Back Cover (Autodesk Fusion 360 design; units mm, degrees)
Autodesk Fusion 360 part; units mm, degrees
sketch "Sketch1" plane through (0, 0, 0) normal (0, 0, 1) x (1, 0, 0)
  line L0 (-79.25, 60.9) -> (79.25, 60.9)
  line L1 (79.25, 60.9) -> (79.25, -60.9)
  line L2 (79.25, -60.9) -> (-79.25, -60.9)
  line L3 (-79.25, -60.9) -> (-79.25, 60.9)
  line L4 (-79.25, 60.9) -> (79.25, -60.9) construction
  line L5 (79.25, 60.9) -> (-79.25, -60.9) construction
  line L6 (79.25, -40.9) -> (-79.25, -40.9)
  line L7 (-79.25, -40.9) -> (-79.25, 40.9)
  line L8 (-79.25, 40.9) -> (79.25, 40.9)
  line L9 (79.25, 40.9) -> (79.25, -40.9)
  line L10 (79.25, -40.9) -> (-79.25, 40.9) construction
  line L11 (-79.25, -40.9) -> (79.25, 40.9) construction
  line L12 (0, 0) -> (0, 60.9) construction
  line L13 (-79.25, 60.9) -> (79.25, 40.9) construction
  line L14 (0, 50.9) -> (-79.25, 50.9) construction
  line L15 (0, 50.9) -> (79.25, 50.9) construction
  line L16 (-2.1, 52.15) -> (-2.1, 49.65)
  arc A0 (-2.1, 49.65) -> (2.1, 49.65) centre (0, 49.65) ccw
  line L17 (2.1, 49.65) -> (2.1, 52.15)
  arc A1 (2.1, 52.15) -> (-2.1, 52.15) centre (0, 52.15) ccw
  line L18 (0, 52.15) -> (0, 49.65) construction
  arc A2 (-50.7333, 52.15) -> (-54.9333, 52.15) centre (-52.8333, 52.15) ccw
  line L19 (-54.9333, 52.15) -> (-54.9333, 49.65)
  arc A3 (-54.9333, 49.65) -> (-50.7333, 49.65) centre (-52.8333, 49.65) ccw
  line L20 (-50.7333, 49.65) -> (-50.7333, 52.15)
  arc A4 (54.9333, 52.15) -> (50.7333, 52.15) centre (52.8333, 52.15) ccw
  line L21 (50.7333, 52.15) -> (50.7333, 49.65)
  arc A5 (50.7333, 49.65) -> (54.9333, 49.65) centre (52.8333, 49.65) ccw
  line L22 (54.9333, 49.65) -> (54.9333, 52.15)
  line L23 (-79.25, 0) -> (79.25, 0) construction
  arc A6 (-54.9333, -52.15) -> (-50.7333, -52.15) centre (-52.8333, -52.15) ccw
  line L24 (-54.9333, -52.15) -> (-54.9333, -49.65)
  arc A7 (-50.7333, -49.65) -> (-54.9333, -49.65) centre (-52.8333, -49.65) ccw
  line L25 (-50.7333, -49.65) -> (-50.7333, -52.15)
  arc A8 (-2.1, -52.15) -> (2.1, -52.15) centre (0, -52.15) ccw
  line L26 (-2.1, -52.15) -> (-2.1, -49.65)
  line L27 (2.1, -49.65) -> (2.1, -52.15)
  arc A9 (2.1, -49.65) -> (-2.1, -49.65) centre (0, -49.65) ccw
  arc A10 (50.7333, -52.15) -> (54.9333, -52.15) centre (52.8333, -52.15) ccw
  line L28 (50.7333, -52.15) -> (50.7333, -49.65)
  line L29 (54.9333, -49.65) -> (54.9333, -52.15)
  arc A11 (54.9333, -49.65) -> (50.7333, -49.65) centre (52.8333, -49.65) ccw
  line L30 (-2.1, 50.9) -> (2.1, 50.9) construction
  line L31 (-37.25, 40.9) -> (-37.25, -40.9) construction
  line L32 (-40.25, 15) -> (-76.25, 15)
  line L33 (-76.25, 15) -> (-76.25, -15)
  line L34 (-76.25, -15) -> (-40.25, -15)
  line L35 (-40.25, -15) -> (-40.25, 15)
  line L36 (-40.25, 15) -> (-76.25, -15) construction
  line L37 (-76.25, 15) -> (-40.25, -15) construction
  line L38 (-43.25, -30) -> (-73.25, -30) construction
  line L39 (-73.25, -30) -> (-73.25, 30) construction
  line L40 (-73.25, 30) -> (-43.25, 30) construction
  line L41 (-43.25, 30) -> (-43.25, -30) construction
  line L42 (-43.25, -30) -> (-73.25, 30) construction
  line L43 (-73.25, -30) -> (-43.25, 30) construction
  circle A12 centre (-73.25, -30) radius 2.1
  circle A13 centre (-43.25, -30) radius 2.1
  circle A14 centre (-73.25, 30) radius 2.1
  circle A15 centre (-43.25, 30) radius 2.1
  line L44 (-79.25, 60.9) -> (-82.25, 60.9)
  line L45 (-82.25, 60.9) -> (-82.25, -60.9)
  line L46 (-82.25, -60.9) -> (-79.25, -60.9)
  line L47 (-79.25, -60.9) -> (-79.25, 60.9)
  point P0 (-58.25, 0)
  point P1 (-58.25, 0)
  dimension "d1" = 121.8
  dimension "d2" = 158.5
  dimension "d3" = 81.8
  dimension "d13" = 4.2
  dimension "d14" = 2.5
  dimension "d22" = 52.8333
  dimension "d23" = 0
  dimension "d26" = 42
  dimension "d27" = 36
  dimension "d28" = 30
  dimension "d29" = 3
  dimension "d30" = 30
  dimension "d31" = 60
  dimension "d32" = 4.2
  dimension "d33" = 4.2
  dimension "d34" = 4.2
  dimension "d35" = 4.2
  dimension "d40" = 3
  constraint perpendicular L0 L1
  constraint parallel L0 L2
  constraint perpendicular L6 L7
  constraint parallel L6 L8
  constraint horizontal L6
  constraint coincident L1 L6.start
  constraint midpoint L0 L12.end
  constraint midpoint L13 L14.start
  constraint coincident L3 L14.end
  constraint perpendicular L3 L14
  constraint coincident L1 L15.end
  constraint perpendicular L1 L15
  constraint tangent L16 A0
  constraint tangent A0 L17
  constraint parallel L16 L17
  constraint tangent L17 A1
  constraint tangent L16 A1
  constraint perpendicular L14 L18
  constraint coincident L12.start L4
  constraint midpoint L12.start L4
  constraint midpoint L12.start L5
  constraint midpoint L12.start L10
  constraint midpoint L12.start L11
  constraint coincident L12.start origin
  constraint coincident L12 A1.centre
  constraint midpoint L3 L23.start
  constraint midpoint L1 L23.end
  constraint symmetric L16.start L23 A8.start
  constraint symmetric L16.end L23 L26.end
  constraint symmetric A0.end L23 L27.start
  constraint symmetric L17.end L23 A8.end
  constraint symmetric A0 L23 A9
  constraint symmetric A1 L23 A8
  constraint symmetric A2.start L23 A6.end
  constraint symmetric A2.end L23 A6.start
  constraint symmetric A2 L23 A6
  constraint symmetric L19.end L23 L24.end
  constraint symmetric A3.end L23 A7.start
  constraint symmetric A3 L23 A7
  constraint symmetric A4.start L23 A10.end
  constraint symmetric A4.end L23 A10.start
  constraint symmetric A4 L23 A10
  constraint symmetric L21.end L23 L28.end
  constraint symmetric A5.end L23 L29.start
  constraint symmetric A5 L23 A11
  constraint midpoint L16 L30.start
  constraint midpoint L17 L30.end
  constraint coincident L14.start L30
  constraint coincident L8 L31.start
  constraint coincident L6 L31.end
  constraint perpendicular L6 L31
  constraint horizontal L32
  constraint perpendicular L32 L33
  constraint parallel L32 L34
  constraint parallel L33 L35
  constraint coincident L36 P1
  constraint coincident L37 P1
  constraint coincident L23 P1
  constraint horizontal L38
  constraint perpendicular L38 L39
  constraint parallel L38 L40
  constraint parallel L39 L41
  constraint coincident L42 P1
  constraint coincident L43 P1
  constraint coincident P1 P0
  constraint coincident L38.end L39.start
  constraint coincident L38.start L41.end
  constraint coincident L39.end L40.start
  constraint coincident L40.end L41.start
  constraint horizontal L44
  constraint vertical L45
  constraint horizontal L46
  constraint vertical L47
  constraint coincident L2.end L3.start
  measures "d1" distance of L0.start L2.end
  measures "d2" distance of L0.start L0.end
  measures "d3" distance of L6.end L7.end
  measures "d13" diameter of A0
  measures "d14" distance of A1.centre A0.centre
  measures "d26" distance of L3 L31
  measures "d27" distance of L33.end L34.end
  measures "d28" distance of L32.end L33.end
  measures "d29" distance of L3 L33
  measures "d30" distance of L39.end L40.end
  measures "d31" distance of L38.end L39.end
  measures "d32" diameter of A12
  measures "d33" diameter of A13
  measures "d34" diameter of A14
  measures "d35" diameter of A15
  measures "d40" distance of L45.end L2.end
extrude "Extrude1" add sketch "Sketch1" along normal blind 9.9 contours L1 L3 L6 L7 L8 L9 L47
extrude "Extrude2" add sketch "Sketch1" against normal blind 3
sketch "Sketch7" plane through (0, 0, 9.9) normal (0, 0, 1) x (-1, 0, 0)
  circle A0 centre (73.25, -30) radius 2.1
  circle A1 centre (43.25, -30) radius 2.1
  circle A2 centre (43.25, 30) radius 2.1
  line L0 (40.25, -15) -> (40.25, 15)
  line L1 (40.25, 15) -> (76.25, 15)
  line L2 (76.25, 15) -> (76.25, -15)
  line L3 (76.25, -15) -> (40.25, -15)
  circle A3 centre (73.25, 30) radius 2.1
  line L4 (-79.25, -40.9) -> (79.25, -40.9)
  line L5 (79.25, -40.9) -> (79.25, 40.9)
  line L6 (79.25, 40.9) -> (-79.25, 40.9)
  line L7 (-79.25, 40.9) -> (-79.25, -40.9)
  line L8 (76.25, -15) -> (79.25, -15)
  line L9 (79.25, -15) -> (79.25, 15)
  line L10 (79.25, 15) -> (76.25, 15)
  line L11 (76.25, 15) -> (76.25, -15)
  constraint horizontal L8
  constraint vertical L9
  constraint horizontal L10
  constraint vertical L11
  constraint coincident L5 L9.end
  constraint coincident L2.end L3.start
extrude "Extrude5" add sketch "Sketch7" along normal blind 5 contours L2 L5 L8 L9 L10 L11
fillet "Fillet1" radius 15 2 edges at (-77.75, 15, 14.9) (-77.75, -15, 14.9)
sketch "Sketch6" plane through (-79.25, 0, 0) normal (-1, 0, 0) x (0, -1, 0)
  line L0 (40.9, 0) -> (40.9, 9.9)
  line L1 (-15, 9.9) -> (-40.9, 9.9)
  line L2 (-40.9, 9.9) -> (-40.9, 0)
  line L3 (-40.9, 0) -> (40.9, 0)
  line L4 (0, 0) -> (0, 10) construction
  circle A0 centre (0, 10) radius 2.1
  arc A1 (15, 9.9) -> (3.8197, 14.9) centre (3.8197, -0.1) ccw
  line L5 (3.8197, 14.9) -> (-3.8197, 14.9)
  arc A2 (-3.8197, 14.9) -> (-15, 9.9) centre (-3.8197, -0.1) ccw
  line L6 (40.9, 9.9) -> (15, 9.9)
  dimension "d36" = 10
  dimension "d37" = 4.2
  constraint coincident L4.start origin
  constraint vertical L4
  constraint coincident L4.end A0.centre
  measures "d36" distance of L4.start L4.end
  measures "d37" diameter of A0
extrude "Extrude4" cut sketch "Sketch6" against normal blind 6 contours A0
equation "d2 = ( 317 / 2 ) * 1 mm"
equation "d22 = ( 158.5 / 3 ) * 1 mm"
equation "d26 = 45 mm - 3 mm"
